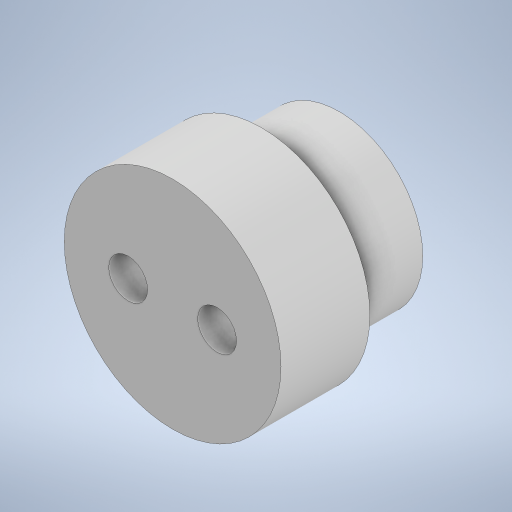
# Autodesk Inventor part: Shaft-1
Saved by Autodesk Inventor 2023 (Build 270158000, 158)
## iProperties
Created: 2023-01-17
Part Number: Shaft-1
Material: Generic
Document SubType Name: Modeling
Designer: caden
Density: 1 g/cm^3
Appearance: Default
Description: 3D Print
Author: caden
Autodesk Inventor part; units mm, degrees
ref_plane "YZ Plane" through (0, 0, 0) normal (1, 0, 0) x (0, 1, 0)
ref_plane "XZ Plane" through (0, 0, 0) normal (0, 1, 0) x (-1, 0, 0)
ref_plane "Work Plane1" through (-12, -12, -7.9972) normal (0, 0, 1) x (1, 0, 0)
sketch "Sketch1" plane through (0, 0, 0) normal (0, 0, 1) x (1, 0, 0)
  circle A0 centre (0, 0) radius 9.75
  circle A1 centre (0, 0) radius 7.5
  dimension "d0" = 19.5
  dimension "d1" = 15
  constraints: 2 centre point, 2 coincident
  measures "d0" diameter of A0
  measures "d1" diameter of A1
extrude "Extrusion1" add sketch "Sketch1" against normal up to surface (7.9972 mm away) contours A0 | A1
extrude "Extrusion2" add sketch "Sketch1" against normal blind 15 contours A1
sketch "Sketch2" plane through (0, 0, -15) normal (0, 0, -1) x (-1, 0, 0)
  circle A0 centre (4, 0) radius 1.75
  circle A1 centre (-4, 0) radius 1.75
  point P0 (0, 0)
  dimension "d6" = 3.5
  dimension "d7" = 4
  dimension "d8" = 8
  constraints: 2 centre point, 1 equal radius
  measures "d6" diameter of A0
  measures "d7" distance of A0.centre point (0, 0)
  measures "d8" distance of A0.centre A1.centre
extrude "Extrusion3" cut sketch "Sketch2" against normal through all
equation "\"d8\" = 2 * d7"
body "Solid1"
